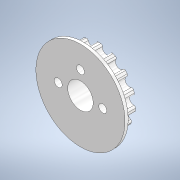
# Autodesk Inventor part: プーリ_歯数15_2.5mm
Saved by Autodesk Inventor 2021 (Build 250183000, 183)
## iProperties
Created: 2022-01-31
Part Number: プーリ_歯数15_2.5mm
Material: アセタール樹脂、白
Document SubType Name: Modeling
Designer: hirohumi
Density: 1.425 g/cm^3
Appearance: 滑らか - 白
Author: hirohumi
Autodesk Inventor part; units mm, degrees
ref_plane "YZ Plane" through (0, 0, 0) normal (1, 0, 0) x (0, 1, 0)
ref_plane "XZ Plane" through (0, 0, 0) normal (0, 1, 0) x (-1, 0, 0)
ref_plane "XY Plane" through (0, 0, 0) normal (0, 0, 1) x (1, 0, 0)
sketch "スケッチ1" plane through (0, 0, 0) normal (0, 0, 1) x (1, 0, 0)
  arc A0 (0.7632, 11.9121) -> (-1.0179, 11.893) centre (0, 0) ccw construction
  arc A1 (0.4062, 11.3607) -> (-0.4062, 11.3607) centre (0, 0) ccw
  arc A2 (9.3048, 1.5803) -> (-9.0567, 2.6555) centre (0, 0) ccw construction
  arc A3 (0.8923, 10.7753) -> (1.9623, 9.2318) centre (2.2471, 10.5718) ccw
  line L0 (1.9623, 9.2318) -> (0, 0)
  arc A4 (-1.9623, 9.2318) -> (-0.8923, 10.7753) centre (-2.2471, 10.5718) ccw
  line L1 (-1.9623, 9.2318) -> (0, 0)
  arc A5 (-0.4062, 11.3607) -> (-0.8923, 10.7753) centre (-0.388, 10.8511) ccw
  arc A6 (0.8923, 10.7753) -> (0.4062, 11.3607) centre (0.388, 10.8511) ccw
  line L2 (0, 0) -> (0, 2.9942) construction
  dimension "d0" = 11.9365
  dimension "d1" = 11.368
  dimension "d2" = 1.93
  dimension "d3" = 0.51
  dimension "d4" = 1.37
  dimension "d5" = 1.37
  dimension "d6" = 24
  dimension "d7" = 12
  constraints: 16 point on circle, 7 centre point, 6 end point, 6 tangent, 3 coincident, 1 equal radius, 1 vertical
  measures "d0" radius of A0
  measures "d1" radius of A1
  measures "d2" radial gap between concentric circles of A2 A1
  measures "d3" radius of A5
  measures "d4" radius of A3
  measures "d5" radius of A4
  measures "d6" angle of L0 L1
  measures "d7" angle of L1 L2
extrude "押し出し1" add sketch "スケッチ1" along normal blind 5
pattern_circular "円形状パターン1" count 15 over 360 about axis through (0, 0, 0) along (0, 0, 1) of "押し出し1"
sketch "スケッチ2" plane through (0, 0, 5) normal (0, 0, 1) x (1, 0, 0)
  circle A0 centre (0, 0) radius 14
  dimension "d13" = 28
  constraints: 1 centre point, 1 coincident
  measures "d13" diameter of A0
extrude "押し出し2" add sketch "スケッチ2" along normal blind 1
sketch "スケッチ3" plane through (0, 0, 0) normal (0, 0, -1) x (-1, 0, 0)
  circle A0 centre (0, 0) radius 4
  circle A1 centre (0, 7) radius 1.25
  circle A2 centre (-7, 0) radius 1.25
  circle A3 centre (7, 0) radius 1.25
  dimension "d16" = 8
  dimension "d18" = 2.5
  dimension "d19" = 7
  dimension "d20" = 2.5
  dimension "d21" = 2.5
  dimension "d22" = 7
  dimension "d23" = 7
  constraints: 4 centre point, 2 horizontal alignment, 1 coincident, 1 vertical alignment
  measures "d16" diameter of A0
  measures "d18" diameter of A1
  measures "d19" distance of point (0, 0) A1.centre
  measures "d20" diameter of A2
  measures "d21" diameter of A3
  measures "d22" distance of point (0, 0) A2.centre
  measures "d23" distance of A3.centre point (0, 0)
extrude "押し出し3" cut sketch "スケッチ3" against normal through all
